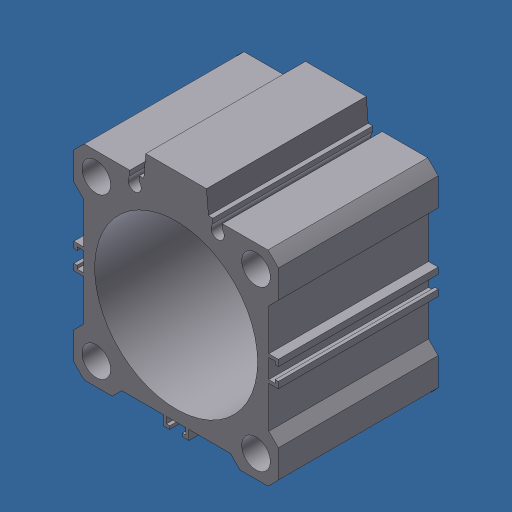
# Autodesk Inventor part: EXTRUSION, CYLINDER, ALUMINIUM, SMC, 50MM
Saved by Autodesk Inventor 2024.3 (Build 283343000, 343)
## iProperties
Manager: _
Category: _
RuleStatus: InUse
Shininess: 64.0
Angle Display Precision: 2
Document Length Units: 11269
Document Angle Units: 11279
Document Time Units: 11290
Document Mass Units: 11283
Document Length Units Precision: 3
Document Angle Units Precision: 2
Part Number: EXTRUSION, CYLINDER, ALUMINIUM, SMC, 50MM
Material: Aluminum, 6061-T6
Document SubType Name: Modeling
Created: 2019-07-31
Designer: -
Manufacturer: Standard
Standards Organization: Custom
Checked By: 00
Engr Approved By: _
User Status: Work In Process
Description: EXTRUSION, CYLINDER, ALUMINIUM, SMC, 50MM
Density: 2.71 g/cm^3
Mass: 213.072 g
Surface Area: 336.233 cm^2
Volume: 78.6243 cm^3
Mfg Approved By: -
Appearance: Aluminum (Flat)
BeforeDocSave0: Mass
BeforeDocSave1: PartFinishTrigger
Density: 0.0
Volumn: 0.0
Area: 0.0
PropertySet Name: Model Information
Control State: 0
Master: False
Checked Out: False
CN_MASS: 0.21
CN_SERVICEABLE: _
CL_runCount: 0
FIRST_DESCRIPTION: _
SECOND_DESCRIPTION: _
THIRD_DESCRIPTION: _
Revision Number: A
Subject: _
Author: -
Keywords: -
Autodesk Inventor part; units mm, degrees
ref_plane "YZ Plane" through (0, 0, 0) normal (1, 0, 0) x (0, 1, 0)
ref_plane "XZ Plane" through (0, 0, 0) normal (0, 1, 0) x (-1, 0, 0)
ref_plane "XY Plane" through (0, 0, 0) normal (0, 0, 1) x (1, 0, 0)
sketch "Sketch1" plane through (0, 0, 0) normal (0, 0, 1) x (1, 0, 0)
  line L0 (0, 60.3133) -> (0, -39.1486) projected
  line L1 (-38.453, 0) -> (51.2707, 0) projected
  line L2 (-32, 28.7228) -> (-32, 20)
  line L3 (-32, 20) -> (-29, 17)
  line L4 (-29, 17) -> (-29, 4)
  line L5 (-29, 4) -> (-32, 4)
  line L6 (-32, 4) -> (-32, 2)
  line L7 (-32, 2) -> (-31, 2)
  line L8 (-31, 2) -> (-31, 3)
  line L9 (-31, 3) -> (-29, 3)
  line L10 (-29, 3) -> (-29, -3)
  line L11 (-29, -3) -> (-31, -3)
  line L12 (-31, -3) -> (-31, -2)
  line L13 (-31, -2) -> (-32, -2)
  line L14 (-32, -2) -> (-32, -4)
  line L15 (-32, -4) -> (-29, -4)
  line L16 (-29, -4) -> (-29, -17)
  line L17 (-29, -17) -> (-32, -20)
  line L18 (-32, -20) -> (-32, -28.7228)
  line L19 (-28.7228, -32) -> (-20, -32)
  line L20 (-20, -32) -> (-17, -29)
  line L21 (-4, -29) -> (-4, -32)
  line L22 (-4, -32) -> (-2, -32)
  line L23 (-2, -32) -> (-2, -31)
  line L24 (-2, -31) -> (-3, -31)
  line L25 (-3, -31) -> (-3, -29)
  line L26 (3, -29) -> (3, -31)
  line L27 (3, -31) -> (2, -31)
  line L28 (2, -31) -> (2, -32)
  line L29 (2, -32) -> (4, -32)
  line L30 (4, -32) -> (4, -29)
  line L31 (17, -29) -> (20, -32)
  line L32 (20, -32) -> (28.7228, -32)
  line L33 (32, -28.7228) -> (32, -20)
  line L34 (32, -20) -> (29, -17)
  line L35 (29, -4) -> (32, -4)
  line L36 (32, -4) -> (32, -2)
  line L37 (32, -2) -> (31, -2)
  line L38 (31, -2) -> (31, -3)
  line L39 (31, -3) -> (29, -3)
  line L40 (31, 3) -> (29, 3)
  line L41 (31, 2) -> (32, 2)
  line L42 (32, 2) -> (32, 4)
  line L43 (32, 4) -> (29, 4)
  line L44 (29, 4) -> (29, 17)
  line L45 (29, 17) -> (32, 20)
  line L46 (32, 20) -> (32, 28.7228)
  line L47 (28.7228, 32) -> (14.5, 32)
  line L48 (14.5, 32) -> (14.5, 30.4337)
  line L49 (11.5, 32) -> (11.5, 30.4337)
  line L50 (10.1124, 32) -> (9.5, 39)
  line L51 (9.5, 39) -> (-9.5, 39)
  line L52 (-9.5, 39) -> (-10.1124, 32)
  line L53 (-11.5, 32) -> (-11.5, 30.4337)
  line L54 (-14.5, 32) -> (-14.5, 30.4337)
  line L55 (31, 3) -> (31, 2)
  arc A0 (-28.7228, 32) -> (-32, 28.7228) centre (0, 0) ccw
  arc A1 (-32, -28.7228) -> (-28.7228, -32) centre (0, 0) ccw
  arc A2 (28.7228, -32) -> (32, -28.7228) centre (0, 0) ccw
  arc A3 (32, 28.7228) -> (28.7228, 32) centre (0, 0) ccw
  line L56 (-17, -29) -> (-4, -29)
  line L57 (17, -29) -> (4, -29)
  line L58 (3, -29) -> (-3, -29)
  line L59 (29, -17) -> (29, -4)
  line L60 (11.5, 32) -> (10.1124, 32)
  line L61 (-14.5, 32) -> (-28.7228, 32)
  arc A4 (-14.5, 30.4337) -> (-11.5, 30.4337) centre (-13, 29) ccw
  arc A5 (11.5, 30.4337) -> (14.5, 30.4337) centre (13, 29) ccw
  line L62 (29, -3) -> (29, 3)
  line L63 (-11.5, 32) -> (-10.1124, 32)
  circle A6 centre (0, 0) radius 25.5
  dimension "d1" = 51
  constraints: 124 end point, 28 vertical, 26 horizontal, 12 point on circle, 7 centre point, 2 point on line, 1 coincident, 1 perpendicular, 14 other
  measures "d1" diameter of A6
extrude "SMC, 50MM" add sketch "Sketch1" against normal blind 50 contours L51 L50 L60 L49 A5 L48 L47 A3 L46 L45 L44 L43 L42 L41 L55 L40 L62 L1 A6 L0 | L0 A6 L1 L10 L9 L8 L7 L6 L5 L4 L3 L2 A0 L61 L54 A4 L53 L63 L52 L51 | L1 L62 L39 L38 L37 L36 L35 L59 L34 L33 A2 L32 L31 L57 L30 L29 L28 L27 L26 L58 L0 A6 | A6 L0 L58 L25 L24 L23 L22 L21 L56 L20 L19 A1 L18 L17 L16 L15 L14 L13 L12 L11 L10 L1
sketch "Sketch2" plane through (0, 0, 0) normal (0, 0, 1) x (1, 0, 0)
  line L0 (0, 60.3) -> (0, -39.1) projected
  line L1 (-38.4, 0) -> (51.2, 0) projected
  point P0 (-25, 25)
  point P1 (-25, -25)
  point P2 (25, -25)
  point P3 (25, 25)
  dimension "d4" = 25
  dimension "d5" = 25
  dimension "d6" = 25
  dimension "d7" = 25
  constraints: 2 horizontal alignment, 2 vertical alignment
  measures "d4" distance from line of point (-25, 25) L0
  measures "d5" distance from line of point (25, 25) L0
  measures "d6" distance from line of point (-25, 25) L1
  measures "d7" distance from line of point (-25, -25) L1
hole "Hole1" at (-25, 25, 0) at (-25, -25, 0) at (25, -25, 0) at (25, 25, 0) direction (0, 0, -1) diameter 9 end through all
equation "\"d5\" = d4"
equation "\"d6\" = d4"
equation "\"d7\" = d4"
